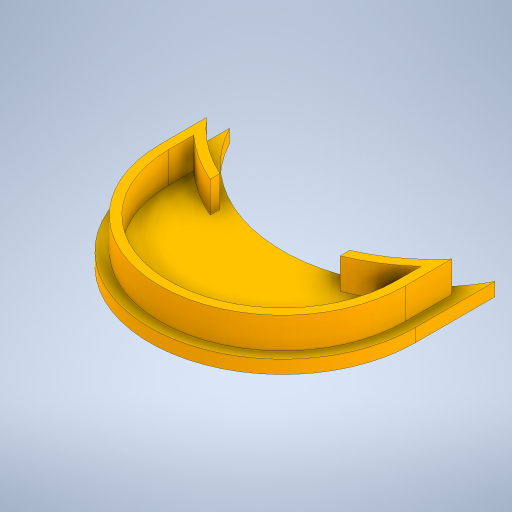
# Autodesk Inventor part: Tapa general
Saved by Autodesk Inventor 2024 (Build 280153000, 153)
## iProperties
Created: 2024-04-29
Part Number: Tapa general
Material: Generic
Document SubType Name: Modeling
Designer: samue
Density: 1 g/cm^3
Appearance: Default
Author: samue
## iProperties of the stored document Tapa general_3DPrint.ipt
Created: 2024-04-29
Part Number: Tapa general_3DPrint
Material: Generic
Document SubType Name: Modeling
Designer: samue
Density: 1 g/cm^3
Appearance: Default
Author: samue
Autodesk Inventor part; units mm, degrees
ref_plane "YZ Plane" through (0, 0, 0) normal (1, 0, 0) x (0, 1, 0)
ref_plane "XZ Plane" through (0, 0, 0) normal (0, 1, 0) x (-1, 0, 0)
ref_plane "XY Plane" through (0, 0, 0) normal (0, 0, 1) x (1, 0, 0)
sketch "Sketch1" plane through (0, 0, 0) normal (0, 1, 0) x (-1, 0, 0)
  arc A0 (30, 0) -> (-30, 0) centre (0, 0) ccw
  line L0 (30, 0) -> (30, -18)
  line L1 (-30, 0) -> (-30, -18)
  arc A1 (30, -18) -> (-30, -18) centre (0, -34) ccw
  dimension "d0" = 60
  dimension "d1" = 34
  dimension "d4" = 18
  constraints: 4 end point, 4 point on circle, 2 centre point, 2 tangent, 2 vertical, 1 coincident, 1 parallel
  measures "d0" diameter of A0
  measures "d1" radius of A1
  measures "d4" distance of L0.start L0.end
extrude "Extrusion1" add sketch "Sketch1" along normal blind 3
sketch "Sketch2" plane through (0, 3, 0) normal (0, 1, 0) x (1, 0, 0)
  arc A0 (-30, 0) -> (30, 0) centre (0, 0) ccw projected
  arc A1 (-30, 18) -> (30, 18) centre (0, 34) ccw projected
  line L0 (-30, 18) -> (-30, 0) projected
  line L1 (30, 0) -> (30, 18) projected
  arc A2 (-27.7, 0) -> (27.7, 0) centre (0, 0) ccw
  line L2 (-27.7, 0) -> (-27.7, 10.5394)
  arc A3 (-27.7, 10.5394) -> (27.7, 10.5394) centre (0, 34) ccw
  line L3 (27.7, 10.5394) -> (27.7, 0)
  arc A4 (-25.7, 0) -> (25.7, 0) centre (0, 0) ccw
  line L4 (-25.7, 0) -> (-25.7, 5.6028)
  arc A5 (-25.7, 5.6028) -> (25.7, 5.6028) centre (0, 34) ccw
  line L5 (25.7, 5.6028) -> (25.7, 0)
  dimension "d5" = 2.3
  dimension "d6" = 2
  constraints: 8 end point, 8 point on circle, 4 centre point, 6 other
  measures "d5" radial gap between concentric circles of A0 A2
  measures "d6" radial gap between concentric circles of A2 A4
extrude "Extrusion2" add sketch "Sketch2" along normal blind 7 contours L2 A3 L3 A2
sketch "Sketch3" plane through (0, 10, 0) normal (0, 1, 0) x (1, 0, 0)
  line L0 (-15.2137, -8.6006) -> (14.4909, -8.6006)
  line L1 (14.4909, -8.6006) -> (14.4909, 18.2853)
  line L2 (14.4909, 18.2853) -> (-15.2137, 18.2853)
  line L3 (-15.2137, 18.2853) -> (-15.2137, -8.6006)
  point P0 (0, 0)
  constraints: 8 end point, 2 parallel, 1 horizontal, 1 perpendicular
extrude "Extrusion3" cut sketch "Sketch3" against normal blind 7
body "Solid1"
